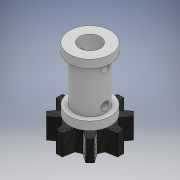
# Autodesk Inventor part: eng_chic_2_1
Saved by Autodesk Inventor 2018 (Build 220112000, 112)
## iProperties
Created: 2018-04-15
Part Number: eng_chic_2_1
Material: Genérico
Document SubType Name: Modeling
Designer: se_ma
Density: 1 g/cm^3
Appearance: Valor por defecto
Author: se_ma
Autodesk Inventor part; units mm, degrees
ref_plane "YZ Plane" through (0, 0, 0) normal (1, 0, 0) x (0, 1, 0)
ref_plane "XZ Plane" through (0, 0, 0) normal (0, 1, 0) x (-1, 0, 0)
ref_plane "XY Plane" through (0, 0, 0) normal (0, 0, 1) x (1, 0, 0)
sketch "Boceto1" plane through (-15.751, -17.109, 5) normal (0, 0, 1) x (1, 0, 0)
  line L0 (0, 0) -> (8.574, 5.146)
  circle A0 centre (4.287, 2.573) radius 4.9998
  point P0 (15.751, 17.109)
  constraints: 2 end point, 1 midpoint, 3 other
extrude "Extrusión1" add sketch "Boceto1" along normal blind 2
sketch "Boceto2" plane through (-11.464, -14.536, 7) normal (0, 0, 1) x (1, 0, 0)
  circle A0 centre (0, 0) radius 3.75
  point P0 (11.464, 14.536)
  dimension "d2" = 7.5
  constraints: 1 centre point
  measures "d2" diameter of A0
extrude "Extrusión2" add sketch "Boceto2" along normal blind 11
sketch "Boceto3" plane through (-11.464, -14.536, 18) normal (0, 0, 1) x (1, 0, 0)
  circle A0 centre (0, 0) radius 4.9998
  point P0 (11.464, 14.536)
  constraints: 1 centre point
extrude "Extrusión3" add sketch "Boceto3" along normal blind 2
sketch "Boceto4" plane through (-11.464, -14.536, 20) normal (0, 0, 1) x (1, 0, 0)
  circle A0 centre (0, 0) radius 2.5
  point P0 (11.464, 14.536)
  dimension "d7" = 5
  constraints: 1 centre point
  measures "d7" diameter of A0
extrude "Extrusión4" cut sketch "Boceto4" against normal blind 22
sketch "Boceto5" plane through (0, 0, 0) normal (1, 0, 0) x (0, 1, 0)
  line L0 (-18.286, 7) -> (-10.786, 7) projected
  line L1 (-14.536, 7) -> (-14.536, 8.5)
  line L2 (-14.536, 8.5) -> (-14.536, 18)
  line L3 (-10.786, 18) -> (-18.286, 18) projected
  line L4 (-14.536, 18) -> (-14.536, 16.5)
  circle A0 centre (-14.536, 16.5) radius 1
  circle A1 centre (-14.536, 8.5) radius 1
  point P0 (0, 0)
  dimension "d10" = 1.5
  dimension "d11" = 1.5
  dimension "d12" = 2
  dimension "d13" = 2
  constraints: 6 end point, 2 centre point, 2 coincident, 2 midpoint, 1 point on line, 1 vertical
  measures "d10" distance of L1.start L1.end
  measures "d11" distance of L2.end L4.end
  measures "d12" diameter of A0
  measures "d13" diameter of A1
extrude "Extrusión5" cut sketch "Boceto5" against normal blind 22
sketch "Boceto7" plane through (-15.751, -17.109, 5) normal (0, 0, 1) x (1, 0, 0)
  circle A0 centre (4.287, 2.573) radius 2.5 projected
  circle A1 centre (4.287, 2.573) radius 2.5
  point P0 (15.751, 17.109)
  constraints: 1 centre point, 1 coincident
extrude "Extrusión6" add sketch "Boceto7" against normal blind 5
sketch "Boceto8" plane through (-11.464, -14.536, 0) normal (0, 0, -1) x (-1, 0, 0)
  circle A0 centre (0, 0) radius 2.5
  point P0 (-11.464, 14.536)
  constraints: 1 centre point
extrude "Extrusión7" cut sketch "Boceto8" against normal blind 5
